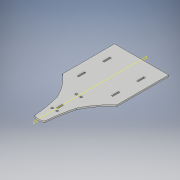
# Autodesk Inventor part: 上底盤新
Saved by Autodesk Inventor 2019 (Build 230136000, 136)
## iProperties
Created: 2020-03-20
Part Number: 上底盤新
Material: Generic
Document SubType Name: Modeling
Designer: 吳昇峻
Density: 1 g/cm^3
Appearance: Default
Author: 吳昇峻
Autodesk Inventor part; units mm, degrees
ref_plane "YZ Plane" through (0, 0, 0) normal (1, 0, 0) x (0, 1, 0)
ref_plane "XZ Plane" through (0, 0, 0) normal (0, 1, 0) x (-1, 0, 0)
ref_plane "XY Plane" through (0, 0, 0) normal (0, 0, 1) x (1, 0, 0)
sketch "Sketch1" plane through (0, 0, 0) normal (0, 1, 0) x (-1, 0, 0)
  line L0 (945.4953, -52.3895) -> (1058.1259, -52.3895)
  arc A0 (945.4953, 55.8486) -> (981.8106, 103.6105) centre (854.964, 162.3701) ccw
  arc A1 (1021.8106, 103.6105) -> (1058.1259, 55.8486) centre (1148.6572, 162.3701) ccw
  line L1 (967.8106, 44.6105) -> (967.8106, 29.6105)
  line L2 (967.8106, -8.3895) -> (967.8106, -23.3895)
  line L3 (967.8106, 44.6105) -> (964.8106, 44.6105)
  line L4 (964.8106, 44.6105) -> (964.8106, 29.6105)
  line L5 (964.8106, 29.6105) -> (967.8106, 29.6105)
  line L6 (967.8106, -23.3895) -> (964.8106, -23.3895)
  line L7 (964.8106, -23.3895) -> (964.8106, -8.3895)
  line L8 (964.8106, -8.3895) -> (967.8106, -8.3895)
  line L9 (1035.8106, 44.6105) -> (1035.8106, 29.6105)
  line L10 (1035.8106, -8.3895) -> (1035.8106, -23.3895)
  line L11 (1035.8106, 44.6105) -> (1038.8106, 44.6105)
  line L12 (1038.8106, 44.6105) -> (1038.8106, 29.6105)
  line L13 (1038.8106, 29.6105) -> (1035.8106, 29.6105)
  line L14 (1035.8106, -23.3895) -> (1038.8106, -23.3895)
  line L15 (1038.8106, -23.3895) -> (1038.8106, -8.3895)
  line L16 (1038.8106, -8.3895) -> (1035.8106, -8.3895)
  line L17 (1058.1259, 55.8486) -> (1058.1259, -52.3895)
  line L18 (945.4953, 55.8486) -> (945.4953, -52.3895)
  line L19 (1001.8106, 123.6105) -> (1003.3106, 123.6105)
  line L20 (1003.3106, 123.6105) -> (1003.3106, 115.6105)
  line L21 (1003.3106, 111.6105) -> (1000.3106, 111.6105)
  line L22 (1000.3106, 115.6105) -> (1000.3106, 123.6257)
  line L23 (1000.3106, 123.6257) -> (1001.8106, 123.6105)
  line L24 (1003.3106, 115.6105) -> (1003.3106, 111.6105)
  line L25 (1000.3106, 115.6105) -> (1000.3106, 111.6105)
  arc A2 (1012.3106, 159.6326) -> (991.3106, 159.6326) centre (1001.8106, 142.6105) ccw
  arc A3 (981.8106, 103.6105) -> (991.3106, 159.6326) centre (700.3575, 180.1548) ccw
  arc A4 (1012.3106, 159.6326) -> (1021.8106, 103.6105) centre (1303.2637, 180.1548) ccw
  arc A5 (945.4953, 55.8486) -> (981.8106, 103.6105) centre (854.964, 162.3701) ccw
  arc A6 (1021.8106, 103.6105) -> (1058.1259, 55.8486) centre (1148.6572, 162.3701) ccw
  line L26 (1001.8106, 123.6105) -> (1003.3106, 123.6105)
  line L27 (1003.3106, 123.6105) -> (1003.3106, 115.6105)
  line L28 (1003.3106, 111.6105) -> (1000.3106, 111.6105)
  line L29 (1000.3106, 115.6105) -> (1000.3106, 123.6105)
  line L30 (1000.3106, 123.6105) -> (1001.8106, 123.6105)
  line L31 (1000.3106, 111.6105) -> (1000.3106, 115.6105)
  line L32 (1003.3106, 111.6105) -> (1003.3106, 115.6105)
  line L33 (1001.8106, 103.6105) -> (1086.8106, 103.6105) construction
  line L34 (1001.8106, 103.6105) -> (916.8106, 103.6105) construction
  line L35 (1086.8106, 133.6105) -> (1071.8106, 133.6105) construction
  line L36 (1071.8106, 133.6105) -> (1071.8106, 73.6105) construction
  line L37 (1071.8106, 73.6105) -> (1101.8106, 73.6105) construction
  line L38 (1101.8106, 73.6105) -> (1101.8106, 133.6105) construction
  line L39 (1101.8106, 133.6105) -> (1086.8106, 133.6105) construction
  line L40 (916.8106, 133.6105) -> (931.8106, 133.6105) construction
  line L41 (931.8106, 133.6105) -> (931.8106, 73.6105) construction
  line L42 (931.8106, 73.6105) -> (901.8106, 73.6105) construction
  line L43 (901.8106, 73.6105) -> (901.8106, 133.6105) construction
  line L44 (901.8106, 133.6105) -> (916.8106, 133.6105) construction
  line L45 (931.8106, 103.6105) -> (935.8106, 103.6105) construction
  line L46 (935.8106, 103.6105) -> (935.8106, 108.6105) construction
  line L47 (1071.8106, 103.6105) -> (1067.8106, 103.6105) construction
  line L48 (1067.8106, 103.6105) -> (1067.8106, 108.6105) construction
  line L49 (935.8106, 103.6105) -> (939.8106, 103.6105) construction
  line L50 (1067.8106, 103.6105) -> (1063.8106, 103.6105) construction
  line L51 (939.8106, 103.6105) -> (949.8106, 103.6105) construction
  line L52 (949.8106, 103.6105) -> (996.7952, 86.5095) construction
  line L53 (949.8106, 103.6105) -> (996.7952, 120.7115) construction
  line L54 (1063.8106, 103.6105) -> (1053.8106, 103.6105) construction
  line L55 (1053.8106, 103.6105) -> (1006.826, 120.7115) construction
  line L56 (1053.8106, 103.6105) -> (1006.826, 86.5095) construction
  line L57 (939.8106, 103.6105) -> (952.4597, 65.6632) construction
  line L58 (952.4597, 65.6632) -> (1051.1615, 65.6632) construction
  line L59 (1051.1615, 65.6632) -> (1063.8106, 103.6105) construction
  line L60 (1001.8106, 123.6105) -> (1001.8106, 168.6105) construction
  line L61 (1001.8106, 123.6105) -> (1003.3106, 123.6105)
  line L62 (1003.3106, 123.6105) -> (1003.3106, 115.6105)
  line L63 (1003.3106, 111.6105) -> (1000.3106, 111.6105)
  line L64 (1000.3106, 115.6105) -> (1000.3106, 123.6257)
  line L65 (1000.3106, 123.6257) -> (1001.8106, 123.6105)
  line L66 (1003.3106, 115.6105) -> (1003.3106, 111.6105)
  line L67 (1000.3106, 115.6105) -> (1000.3106, 111.6105)
  arc A7 (1012.3106, 159.6326) -> (991.3106, 159.6326) centre (1001.8106, 142.6105) ccw
  arc A8 (981.8106, 103.6105) -> (991.3106, 159.6326) centre (700.3575, 180.1548) ccw
  arc A9 (1012.3106, 159.6326) -> (1021.8106, 103.6105) centre (1303.2637, 180.1548) ccw
  line L68 (1001.8106, 78.6105) -> (1006.8106, 78.6105) construction
  line L69 (1006.8106, 78.6105) -> (1006.8106, 128.6105) construction
  line L70 (1006.8106, 128.6105) -> (996.8106, 128.6105) construction
  line L71 (996.8106, 128.6105) -> (996.8106, 78.6105) construction
  line L72 (996.8106, 78.6105) -> (1001.8106, 78.6105) construction
  circle A10 centre (1006.8106, 78.6105) radius 2.25
  circle A11 centre (996.8106, 78.6105) radius 2.25
  circle A12 centre (1006.8106, 128.6105) radius 2.25
  circle A13 centre (996.8106, 128.6105) radius 2.25
  point P0 (0, 0)
  constraints: 146 end point, 20 point on circle, 14 centre point, 12 point on line, 2 midpoint
extrude "Extrusion1" add sketch "Sketch1" along normal blind 3
ref_plane "Work Plane1" through (-1001.8106, 0, 55.8486) normal (1, 0, 0) x (0, 0, -1)
body "Solid1"
